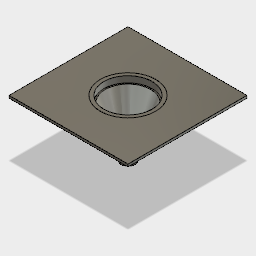
Yogurt Funnel v0 (Autodesk Fusion 360 design; units mm, degrees)
Autodesk Fusion 360 part; units mm, degrees
note: some values were not read from the file. Chosen so that the rebuilt part matches the saved one: which bodies a step acts on.
sketch "Sketch1" plane through (0, 0, 0) normal (0, 0, 1) x (1, 0, 0)
  line L0 (0.2702, 60.256) -> (0.2702, 0.256)
  line L1 (0.2702, 0.256) -> (22.1084, 60.256)
  line L2 (22.1084, 60.256) -> (0.2702, 60.256)
  dimension "d1" = 20
  dimension "d2" = 90
  measures "d1" angle of L0 L1
  measures "d2" angle of L0 L2
revolve "Revolve1" add sketch "Sketch1" angle 360 about axis through (0, 1.75, 0) along (0, 1, 0) makes body 1
ref_plane "WorkPlane1" through (0, 60.256, 0) normal (0, 1, 0) x (0, 0, 1)
sketch "Sketch2" plane through (0, 60.256, 0) normal (0, 1, 0) x (1, 0, 0)
shell "Shell1" thickness 2 removed faces 0 bodies 1
ref_plane "WorkPlane2" through (0, 60.256, 0) normal (0, 1, 0) x (0, 0, 1)
sketch "Sketch3" plane through (0, 60.256, 0) normal (0, 1, 0) x (1, 0, 0)
  line L0 (-47.625, 47.625) -> (47.625, 47.625)
  line L1 (47.625, 47.625) -> (47.625, -47.625)
  line L2 (47.625, -47.625) -> (-47.625, -47.625)
  line L3 (-47.625, -47.625) -> (-47.625, 47.625)
  circle A0 centre (0, 0) radius 22.1084
  circle A1 centre (0, 0) radius 22.1084
  point P0 (0, 47.625)
  point P1 (-47.625, 0)
  dimension "d7" = 95.25
  dimension "d8" = 95.25
  measures "d7" distance of L0.start L0.end
  measures "d8" distance of L0.start L2.end
extrude "Extrude1" add sketch "Sketch3" against normal blind 2 bodies 1
sketch "Sketch4" plane through (0, 60.256, 0) normal (0, 1, 0) x (-1, 0, 0)
  circle A0 centre (0, 0) radius 0.2702
  circle A1 centre (0, 0) radius 22.1084
  circle A2 centre (0, 0) radius 20.1084
  circle A3 centre (0, 0) radius 19.2521
  dimension "d11" = 2
  measures "d11" distance of A1 A2
extrude "Extrude2" cut sketch "Sketch4" against normal blind 5 contours A3 bodies 1
sketch "Sketch5" plane through (0, 0, 0) normal (1, 0, 0) x (0, 0, -1)
  line L0 (25, 15) -> (-35, 15)
split "Split1" by curves path "Sketch5" along L0 bodies 1 makes body 3 at (0.5507, 60.256, -39.0989) makes body 3 at (-7.0741, 52.7134, 18.0246) makes body 2 at (2.2673, 41.8374, -0.1132)
hidden bodies 1 2
